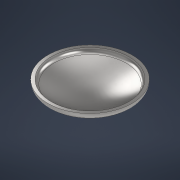
# Autodesk Inventor part: tank endcap
Saved by Autodesk Inventor 2021 (Build 250183000, 183)
## iProperties
Created: 2020-12-02
Part Number: tank endcap
Material: Stainless Steel
Document SubType Name: Modeling
Designer: henry
Density: 8 g/cm^3
Appearance: Semi-Polished
Mass: 57.4591 g
Surface Area: 55.6809 cm^2
Volume: 7.18239 cm^3
Author: henry
Autodesk Inventor part; units mm, degrees
ref_plane "YZ Plane" through (0, 0, 0) normal (1, 0, 0) x (0, 1, 0)
ref_plane "XZ Plane" through (0, 0, 0) normal (0, 1, 0) x (-1, 0, 0)
ref_plane "XY Plane" through (0, 0, 0) normal (0, 0, 1) x (1, 0, 0)
sketch "ox tank wall cross section" plane through (0, 135.9717, 0) normal (0, 1, 0) x (-1, 0, 0)
  circle A0 centre (0, 0) radius 25
  circle A1 centre (0, 0) radius 27
  point P0 (-25, 0)
sketch "end cap profile" plane through (0, 0, 0) normal (0, 0, 1) x (1, 0, 0)
  line L0 (25, 135.9717) -> (-25, 135.9717) construction
  line L1 (27, 135.9717) -> (-27, 135.9717) projected
  arc A0 (24.8893, 131.891) -> (27, 135.9717) centre (22, 135.9717) ccw
  arc A1 (0, 123.9717) -> (24.8893, 131.891) centre (0, 167.0431) ccw
  line L2 (0, 123.9717) -> (0, 127.9717)
  line L3 (-27, 135.9717) -> (25, 135.9717) construction
  arc A2 (22, 135.9717) -> (22, 135.9717) centre (22, 135.9717) ccw construction
  line L4 (0, 134.2393) -> (0, 137.2393) construction
  arc A3 (23.2967, 133.2664) -> (25, 135.9717) centre (22, 135.9717) ccw
  arc A4 (0, 127.9717) -> (23.2967, 133.2664) centre (0, 181.8717) ccw
  line L5 (0, 127.9717) -> (0, 135.9717) construction
  line L6 (25, 135.9717) -> (22, 135.9717) construction
  line L7 (0, -36.3743) -> (0, 218.2461) projected
  line L8 (25, 135.9717) -> (27, 135.9717)
  point P0 (0, 0)
  dimension "d7" = 3
  dimension "d9" = 8
  dimension "d11" = 4
  constraints: 12 end point, 10 point on circle, 5 centre point, 5 line through centre, 2 perpendicular, 2 tangent, 1 coincident, 1 collinear, 1 midpoint, 1 point on line
  measures "d7" radius of A3
  measures "d9" distance of L5.end L2.end
  measures "d11" distance of L2.start L2.end
revolve "Revolution1" add sketch "end cap profile" angle 360 about axis through (0, -10, 0) along (0, 1, 0) contours A0 A1 L2 A4 A3 L1
body "Solid4"
